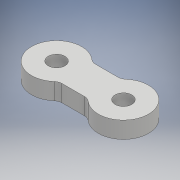
# Autodesk Inventor part: кривошип_v1
Saved by Autodesk Inventor 2017.3 (Build 213256000, 256)
## iProperties
Part Number: кривошип_v1
Material: Типовые
Document SubType Name: Modeling
Designer: Alexnav
Density: 1 g/cm^3
Appearance: По умолчанию
Mass: 15.0658 g
Surface Area: 54.33 cm^2
Volume: 15.0658 cm^3
Author: Alexnav
Autodesk Inventor part; units mm, degrees
ref_plane "YZ Plane" through (0, 0, 0) normal (1, 0, 0) x (0, 1, 0)
ref_plane "XZ Plane" through (0, 0, 0) normal (0, 1, 0) x (-1, 0, 0)
ref_plane "XY Plane" through (0, 0, 0) normal (0, 0, 1) x (1, 0, 0)
sketch "Эскиз1" plane through (0, 0, 0) normal (0, 0, 1) x (1, 0, 0)
  line L0 (-49, 0) -> (49, 0) projected
  line L1 (-6.7712, 10) -> (6.7712, 10)
  line L2 (6.7712, -10) -> (-6.7712, -10)
  line L3 (0, -21) -> (0, 21) projected
  arc A0 (-10.0784, 11.25) -> (-10.0784, -11.25) centre (-20, 0) ccw
  arc A1 (10.0784, -11.25) -> (10.0784, 11.25) centre (20, 0) ccw
  circle A2 centre (-20, 0) radius 5
  circle A3 centre (20, 0) radius 5
  arc A4 (-10.0784, 11.25) -> (-6.7712, 10) centre (-6.7712, 15) ccw
  arc A5 (-6.7712, -10) -> (-10.0784, -11.25) centre (-6.7712, -15) ccw
  arc A6 (10.0784, -11.25) -> (6.7712, -10) centre (6.7712, -15) ccw
  arc A7 (6.7712, 10) -> (10.0784, 11.25) centre (6.7712, 15) ccw
  point P0 (0, 0)
  point P1 (-8.8197, 10)
  point P2 (8.8197, -10)
  point P3 (8.8197, 10)
  point P4 (-8.8197, -10)
  dimension "d1" = 20
  dimension "d3" = 15
  dimension "d4" = 10
  dimension "d5" = 5
  dimension "d8" = 40
  constraints: 16 point on circle, 8 centre point, 8 tangent, 6 point on line, 5 equal radius, 4 end point, 2 coincident, 2 parallel, 2 symmetric about line, 1 horizontal, 1 other
  measures "d1" distance of point (8.82, 10) point (8.82, -10)
  measures "d3" radius of A0
  measures "d4" diameter of A2
  measures "d5" radius of A4
  measures "d8" distance of A3.centre A0.centre
extrude "Выдавливание1" add sketch "Эскиз1" along normal blind 10
sketch "Эскиз2" plane through (0, 0, 0) normal (0, 0, -1) x (-1, 0, 0)
  circle A0 centre (-20, 0) radius 5 projected
  point P0 (0, 0)
extrude "Выдавливание2" cut sketch "Эскиз2" along normal through all both and the other way through all
sketch "Эскиз3" plane through (0, 0, 10) normal (0, 0, 1) x (1, 0, 0)
  circle A0 centre (-20, 0) radius 5 projected
  point P0 (0, 0)
extrude "Выдавливание3" cut sketch "Эскиз3" along normal through all both and the other way through all
